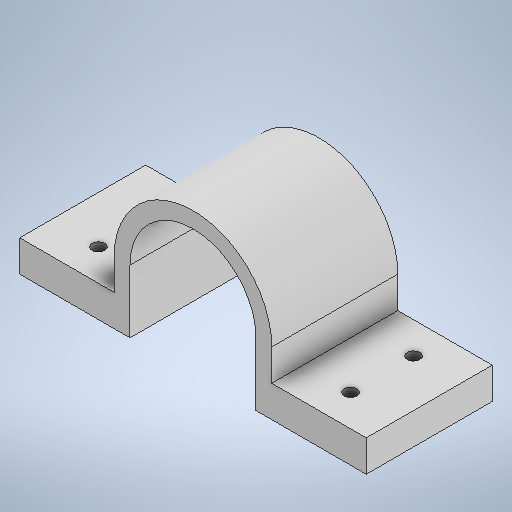
# Autodesk Inventor part: U-bracket
Saved by Autodesk Inventor 2025.3 (Build 293356030, 356C)
## iProperties
Created: 2026-06-26
Part Number: U-bracket
Material: Generic
Document SubType Name: Modeling
Designer: user
Density: 1 g/cm^3
Appearance: Default
Author: user
Autodesk Inventor part; units mm, degrees
ref_plane "YZ Plane" through (0, 0, 0) normal (1, 0, 0) x (0, 1, 0)
ref_plane "XZ Plane" through (0, 0, 0) normal (0, 1, 0) x (-1, 0, 0)
ref_plane "XY Plane" through (0, 0, 0) normal (0, 0, 1) x (1, 0, 0)
sketch "Sketch1" plane through (0, 0, 0) normal (0, 0, 1) x (1, 0, 0)
  arc A0 (20, 20) -> (-20, 20) centre (0, 20) ccw
  line L0 (55, 0) -> (55, 10)
  line L1 (-55, 10) -> (-55, 0)
  line L2 (55, 10) -> (25, 10)
  line L3 (-25, 10) -> (-55, 10)
  line L4 (20, 20) -> (20, 0)
  line L5 (-20, 20) -> (-20, 0)
  line L6 (25, 20) -> (25, 10)
  line L7 (-25, 20) -> (-25, 10)
  arc A1 (25, 20) -> (-25, 20) centre (0, 20) ccw
  line L8 (-55, 0) -> (-20, 0)
  line L9 (20, 0) -> (55, 0)
  point P0 (0, 0)
  dimension "d1" = 10
  dimension "d4" = 55
  dimension "d5" = 30
  dimension "d6" = 30
  dimension "d7" = 55
  constraints: 20 end point, 5 parallel, 5 point on circle, 4 perpendicular, 3 tangent, 2 centre point, 2 horizontal, 1 coincident
  measures "d1" distance of L0.end L0.start
  measures "d4" horizontal distance of L0.end A0.centre
  measures "d5" distance of L0.end L2.end
  measures "d6" distance of L3.start L1.start
  measures "d7" distance from line of L1 A0.centre
extrude "Extrusion1" add sketch "Sketch1" along normal blind 40
sketch "Sketch2" plane through (25, 10, 0) normal (0, 1, 0) x (1, 0, 0)
  point P0 (-25, 0)
sketch "Sketch3" plane through (25, 10, 0) normal (0, 1, 0) x (1, 0, 0)
  line L0 (30, 0) -> (0, 0) construction
  line L1 (15, 0) -> (15, -40) construction
  line L2 (30, -40) -> (0, -40) construction
  line L3 (30, 0) -> (30, -40) construction
  line L4 (30, -20) -> (-80, -20) construction
  line L5 (-80, 0) -> (-80, -40) construction
  line L6 (-50, 0) -> (-80, 0) construction
  line L7 (-65, 0) -> (-65, -40) construction
  line L8 (-50, -40) -> (-80, -40) construction
  line L9 (-80, -10) -> (30, -10) construction
  line L10 (-80, -30) -> (30, -30) construction
  circle A0 centre (15, -10) radius 2
  circle A1 centre (15, -30) radius 2
  circle A2 centre (-65, -10) radius 2
  circle A3 centre (-65, -30) radius 2
  point P0 (-25, 0)
  dimension "d8" = 4
  dimension "d9" = 4
  dimension "d10" = 4
  dimension "d11" = 4
  constraints: 10 end point, 10 point on line, 6 midpoint, 4 centre point, 1 horizontal, 1 perpendicular
  measures "d8" diameter of A0
  measures "d9" diameter of A1
  measures "d10" diameter of A2
  measures "d11" diameter of A3
extrude "Extrusion2" cut sketch "Sketch3" against normal blind 10
thread "Thread1" size "M4x0.7" class "6H" standard "ISO Metric profile" length 150
thread "Thread2" size "M4x0.7" class "6H" standard "ISO Metric profile" length 150
thread "Thread3" size "M4x0.7" class "6H" standard "ISO Metric profile" length 150
thread "Thread4" size "M4x0.7" class "6H" standard "ISO Metric profile" length 150
body "Solid1"
